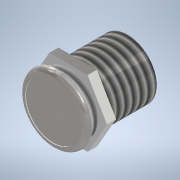
# Autodesk Inventor part: Button
Saved by Autodesk Inventor 2021 (Build 250183000, 183)
## iProperties
Created: 2022-09-01
Part Number: Button
Material: Generic
Document SubType Name: Modeling
Designer: cmzgt
Density: 1 g/cm^3
Appearance: Default
Author: cmzgt
Autodesk Inventor part; units mm, degrees
ref_plane "YZ Plane" through (0, 0, 0) normal (1, 0, 0) x (0, 1, 0)
ref_plane "XZ Plane" through (0, 0, 0) normal (0, 1, 0) x (-1, 0, 0)
sketch "Sketch3" plane through (0, 0, 0) normal (0, 0, 1) x (1, 0, 0)
  circle A0 centre (0, 0) radius 9.5
  dimension "d3" = 19
  constraints: 1 centre point, 1 coincident
  measures "d3" diameter of A0
extrude "Extrusion2" add sketch "Sketch3" along normal blind 22.4
sketch "Sketch4" plane through (0, 0, 22.4) normal (0, 0, 1) x (1, 0, 0)
  circle A0 centre (0, 0) radius 10.95
  dimension "d6" = 21.9
  constraints: 1 centre point, 1 coincident
  measures "d6" diameter of A0
extrude "Extrusion3" add sketch "Sketch4" along normal blind 2
sketch "Sketch5" plane through (0, 0, 24.4) normal (0, 0, 1) x (1, 0, 0)
  circle A0 centre (0, 0) radius 8.89
  dimension "d10" = 17.78
  constraints: 1 centre point, 1 coincident
  measures "d10" diameter of A0
fillet "Fillet1" radius 1.905 1 edges at (-10.95, 0, 24.4)
ref_plane "Work Plane3" through (0, 0, 19.2) normal (0, 0, -1) x (-1, 0, 0)
sketch "Sketch6" plane through (0, 0, 19.2) normal (0, 0, -1) x (-1, 0, 0)
  line L0 (6.2278, -10.8381) -> (-6.2721, -10.8125)
  line L1 (-6.2721, -10.8125) -> (-12.5, 0.0256)
  line L2 (-12.5, 0.0256) -> (-6.2278, 10.8381)
  line L3 (-6.2278, 10.8381) -> (6.2721, 10.8125)
  line L4 (6.2721, 10.8125) -> (12.5, -0.0256)
  line L5 (12.5, -0.0256) -> (6.2278, -10.8381)
  point P0 (0, 0)
  point P1 (0, 0)
  dimension "d13" = 25
  dimension "d14" = 10.8125
  constraints: 12 end point, 1 coincident, 13 other
  measures "d13" distance of L2.end L0.start
  measures "d14" vertical distance of L4.end L0.start
extrude "Extrusion4" add sketch "Sketch6" along normal blind 3
extrude "Extrusion5" cut sketch "Sketch5" against normal blind 0.225
thread "Thread2" size "M20x2.5" class "6g" standard "ANSI Metric M Profile" length 25.4
body "Solid2"
